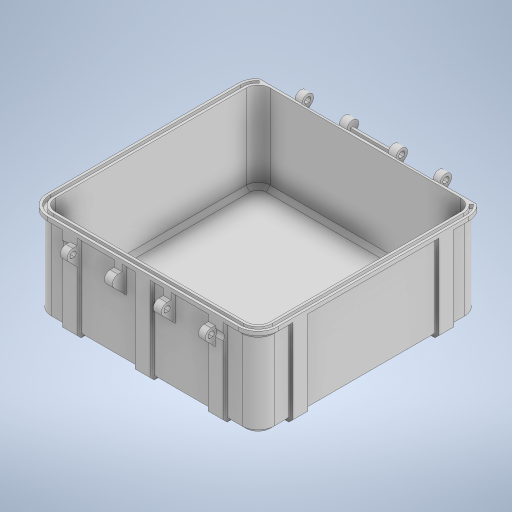
# Autodesk Inventor part: universal_box-main_body
Saved by Autodesk Inventor 2024 (Build 280153000, 153)
## iProperties
Created: 2024-03-05
Part Number: universal_box-main_body
Material: Všeobecné
Document SubType Name: Modeling
Designer: Simak
Density: 1 g/cm^3
Appearance: Výchozí
Author: Simak
Autodesk Inventor part; units mm, degrees
ref_plane "YZ Plane" through (0, 0, 0) normal (1, 0, 0) x (0, 1, 0)
ref_plane "XZ Plane" through (0, 0, 0) normal (0, 1, 0) x (-1, 0, 0)
ref_plane "XY Plane" through (0, 0, 0) normal (0, 0, 1) x (1, 0, 0)
sketch "velikost" plane through (0, 0, 0) normal (0, 1, 0) x (-1, 0, 0)
  line L0 (55.5, -55.5) -> (-55.5, -55.5)
  line L1 (-55.5, -55.5) -> (-55.5, 55.5)
  line L2 (-55.5, 55.5) -> (55.5, 55.5)
  line L3 (55.5, 55.5) -> (55.5, -55.5)
  line L4 (55.5, -55.5) -> (0, 0) construction
  line L5 (0, 0) -> (-55.5, -55.5) construction
  line L6 (0, 0) -> (-55.5, 55.5) construction
  dimension "d0" = 111
  dimension "d1" = 111
  constraints: 14 end point, 2 equal length, 2 parallel, 1 horizontal, 1 perpendicular
  measures "d0" distance of L0.start L0.end
  measures "d1" distance of L0.end L1.end
extrude "vyska" add sketch "velikost" along normal blind 46
fillet "Zaobleni_rohu" radius 8 4 edges at (-55.5, 23, 55.5) (55.5, 23, 55.5) (55.5, 23, -55.5) (-55.5, 23, -55.5)
shell "tloustka_sten" thickness 2 removed faces 1 at (15.8333, 46, -18.5)
sketch "vyztuhy-velikost" plane through (0, 46, 0) normal (0, 1, 0) x (1, 0, 0)
  arc A0 (-47.5, 53.5) -> (-53.5, 47.5) centre (-47.5, 47.5) ccw projected
  line L0 (-47.5, 53.5) -> (47.5, 53.5) projected
  arc A1 (53.5, 47.5) -> (47.5, 53.5) centre (47.5, 47.5) ccw projected
  line L1 (53.5, 47.5) -> (53.5, -47.5) projected
  arc A2 (47.5, -53.5) -> (53.5, -47.5) centre (47.5, -47.5) ccw projected
  line L2 (47.5, -53.5) -> (-47.5, -53.5) projected
  arc A3 (-53.5, -47.5) -> (-47.5, -53.5) centre (-47.5, -47.5) ccw projected
  line L3 (-53.5, -47.5) -> (-53.5, 47.5) projected
  arc A4 (-47.5, 55.5) -> (-55.5, 47.5) centre (-47.5, 47.5) ccw projected
  line L4 (-55.5, 47.5) -> (-55.5, -47.5) projected
  arc A5 (-55.5, -47.5) -> (-47.5, -55.5) centre (-47.5, -47.5) ccw projected
  line L5 (-47.5, -55.5) -> (47.5, -55.5) projected
  arc A6 (47.5, -55.5) -> (55.5, -47.5) centre (47.5, -47.5) ccw projected
  line L6 (55.5, -47.5) -> (55.5, 47.5) projected
  arc A7 (55.5, 47.5) -> (47.5, 55.5) centre (47.5, 47.5) ccw projected
  line L7 (47.5, 55.5) -> (-47.5, 55.5) projected
  line L8 (-40.1, 55.5) -> (-40.1, 57.5)
  line L9 (-40.1, 57.5) -> (-32.7, 57.5)
  line L10 (-32.7, 57.5) -> (-32.7, 55.5)
  line L11 (-3.7, 55.5) -> (-3.7, 57.5)
  line L12 (-3.7, 57.5) -> (3.7, 57.5)
  line L13 (3.7, 57.5) -> (3.7, 55.5)
  line L14 (32.7, 55.5) -> (32.7, 57.5)
  line L15 (32.7, 57.5) -> (40.1, 57.5)
  line L16 (40.1, 57.5) -> (40.1, 55.5)
  line L17 (47.5, 55.5) -> (-47.5, 55.5) projected
  line L18 (-3.7, 57.5) -> (0, 55.5) construction
  line L19 (3.7, 57.5) -> (0, 55.5) construction
  line L20 (-32.7, 57.5) -> (-3.7, 57.5) construction
  line L21 (3.7, 57.5) -> (32.7, 57.5) construction
  line L22 (-40.1, 57.5) -> (-47.5, 57.5) construction
  line L23 (-47.5, 57.5) -> (-47.5, 55.5) construction
  line L24 (-53.5, 0) -> (53.5, 0)
  line L25 (0, 53.5) -> (0, -53.5)
  line L26 (47.5, -53.5) -> (-47.5, -53.5) projected
  line L27 (-55.5, -40.1) -> (-57.5, -40.1)
  line L28 (-57.5, -40.1) -> (-57.5, -32.7)
  line L29 (-57.5, -32.7) -> (-55.5, -32.7)
  line L30 (-55.5, 32.7) -> (-57.5, 32.7)
  line L31 (-57.5, 32.7) -> (-57.5, 40.1)
  line L32 (-57.5, 40.1) -> (-55.5, 40.1)
  line L33 (-57.5, -32.7) -> (-57.5, 32.7) construction
  line L34 (-57.5, -40.1) -> (-57.5, -47.5) construction
  line L35 (-57.5, -47.5) -> (-55.5, -47.5) construction
  line L36 (-55.5, 47.5) -> (-55.5, -47.5) projected
  line L37 (-57.5, 40.1) -> (-57.5, 47.5) construction
  line L38 (-57.5, 47.5) -> (-55.5, 47.5) construction
  line L39 (-55.5, 0) -> (-57.5, 32.7) construction
  line L40 (-55.5, 0) -> (-57.5, -32.7) construction
  line L41 (-40.1, -55.5) -> (-40.1, -57.5)
  line L42 (-40.1, -57.5) -> (-32.7, -57.5)
  line L43 (-32.7, -57.5) -> (-32.7, -55.5)
  line L44 (-3.7, -55.5) -> (-3.7, -57.5)
  line L45 (-3.7, -57.5) -> (3.7, -57.5)
  line L46 (3.7, -57.5) -> (3.7, -55.5)
  line L47 (32.7, -55.5) -> (32.7, -57.5)
  line L48 (32.7, -57.5) -> (40.1, -57.5)
  line L49 (40.1, -57.5) -> (40.1, -55.5)
  line L50 (47.5, -55.5) -> (-47.5, -55.5)
  line L51 (-3.7, -57.5) -> (0, -55.5) construction
  line L52 (3.7, -57.5) -> (0, -55.5) construction
  line L53 (-32.7, -57.5) -> (-3.7, -57.5) construction
  line L54 (3.7, -57.5) -> (32.7, -57.5) construction
  line L55 (-40.1, -57.5) -> (-47.5, -57.5) construction
  line L56 (-47.5, -57.5) -> (-47.5, -55.5) construction
  line L57 (55.5, 47.5) -> (55.5, -47.5)
  line L58 (57.5, -32.7) -> (57.5, 32.7) construction
  line L59 (55.5, -40.1) -> (57.5, -40.1)
  line L60 (57.5, -40.1) -> (57.5, -47.5) construction
  line L61 (57.5, -32.7) -> (55.5, -32.7)
  line L62 (57.5, -47.5) -> (55.5, -47.5) construction
  line L63 (57.5, -40.1) -> (57.5, -32.7)
  line L64 (57.5, 32.7) -> (57.5, 40.1)
  line L65 (57.5, 40.1) -> (55.5, 40.1)
  line L66 (55.5, 32.7) -> (57.5, 32.7)
  line L67 (55.5, 47.5) -> (55.5, -47.5)
  line L68 (57.5, 40.1) -> (57.5, 47.5) construction
  line L69 (57.5, 47.5) -> (55.5, 47.5) construction
  line L70 (55.5, 0) -> (57.5, 32.7) construction
  line L71 (55.5, 0) -> (57.5, -32.7) construction
  point P0 (0, 0)
  point P1 (55.5, 40.1)
  point P2 (55.5, 32.7)
  point P3 (55.5, -32.7)
  point P4 (55.5, -40.1)
  point P5 (40.1, -55.5)
  point P6 (32.7, -55.5)
  point P7 (3.7, -55.5)
  point P8 (-3.7, -55.5)
  point P9 (-32.7, -55.5)
  point P10 (-40.1, -55.5)
  point P11 (-55.5, -40.1)
  point P12 (-55.5, -32.7)
  point P13 (-55.5, 32.7)
  point P14 (-55.5, 40.1)
  dimension "d6" = 2
  dimension "d7" = 7.4
  dimension "d8" = 2
  constraints: 120 end point, 25 symmetric about line, 20 point on line, 14 equal length, 11 perpendicular, 5 midpoint, 5 vertical, 2 horizontal, 5 other
  measures "d6" distance of L9.end L10.end
  measures "d7" distance of L11.end L12.end
  measures "d8" distance of L33.start L29.end
extrude "vyztuhy" add sketch "vyztuhy-velikost" against normal up to surface (46 mm away) contours L8 L9 L10 L7 | L4 L30 L31 L32 | L11 L12 L13 L7 | L4 L27 L28 L29 | L14 L15 L16 L7 | L5 L43 L42 L41 | L65 L64 L66 L6 | L5 L46 L45 L44 | L61 L63 L59 L6 | L5 L49 L48 L47
chamfer "Zkoseni_spodku" distance 2 angle 45 36 edges at (-18.2, 0, 55.5) (18.2, 0, 55.5) (0, 0, 57.5) (36.4, 0, 57.5) (43.8, 0, 55.5) (53.1569, 0, 53.1569) (55.5, 0, 43.8) (57.5, 0, 36.4) (55.5, 0, 0) (57.5, 0, -36.4) (53.1569, 0, -53.1569) (43.8, 0, -55.5) (55.5, 0, -43.8) (36.4, 0, -57.5) (18.2, 0, -55.5) (0, 0, -57.5) (-18.2, 0, -55.5) (-36.4, 0, -57.5) (-43.8, 0, -55.5) (-53.1569, 0, -53.1569) (-55.5, 0, -43.8) (-57.5, 0, -36.4) (-55.5, 0, 0) (-57.5, 0, 36.4) (-55.5, 0, 43.8) (-53.1569, 0, 53.1569) (-43.8, 0, 55.5) (-36.4, 0, 57.5) (-53.5, 2, 0) (-51.7426, 2, 51.7426) (0, 2, 53.5) (51.7426, 2, 51.7426) (53.5, 2, 0) (51.7426, 2, -51.7426) (0, 2, -53.5) (-51.7426, 2, -51.7426)
sketch "Náčrt4" plane through (40.1, 46, -55.5) normal (1, 0, 0) x (0, 0, -1)
  line L0 (-2, 0) -> (-2, -42) projected
  line L1 (2, 0) -> (2, -44) projected
  line L2 (-8, 0) -> (0, 0) projected
  line L3 (-0.75, 0) -> (-0.75, -2)
  line L4 (-0.75, -2) -> (0.75, -2)
  line L5 (0.75, -2) -> (0.75, 0)
  line L6 (-0.75, -2) -> (-2, -2) construction
  line L7 (0.75, -2) -> (2, -2) construction
  line L8 (2, 0) -> (0, 0) projected
  line L9 (2, -4) -> (-2, -4)
  point P0 (-55.5, -46)
  dimension "d16" = 1.5
  dimension "d17" = 2
  dimension "d18" = 2
  constraints: 12 end point, 7 point on line, 5 perpendicular, 1 collinear
  measures "d16" distance of L3.end L4.end
  measures "d17" distance between parallel lines of L8 L4
  measures "d18" distance between parallel lines of L9 L4
sketch "Náčrt3" plane through (0, 46, 0) normal (0, 1, 0) x (1, 0, 0)
  arc A0 (-47.5, 53.5) -> (-53.5, 47.5) centre (-47.5, 47.5) ccw projected
  line L0 (-47.5, 53.5) -> (47.5, 53.5) projected
  arc A1 (53.5, 47.5) -> (47.5, 53.5) centre (47.5, 47.5) ccw projected
  line L1 (53.5, 47.5) -> (53.5, -47.5) projected
  arc A2 (47.5, -53.5) -> (53.5, -47.5) centre (47.5, -47.5) ccw projected
  line L2 (47.5, -53.5) -> (-47.5, -53.5) projected
  arc A3 (-53.5, -47.5) -> (-47.5, -53.5) centre (-47.5, -47.5) ccw projected
  line L3 (-53.5, -47.5) -> (-53.5, 47.5) projected
  arc A4 (-47.5, 55.5) -> (-55.5, 47.5) centre (-47.5, 47.5) ccw projected
  line L4 (-55.5, 47.5) -> (-55.5, 40.1) projected
  line L5 (-57.5, 32.7) -> (-55.5, 32.7) projected
  line L6 (-55.5, 32.7) -> (-55.5, -32.7) projected
  arc A5 (-55.5, -47.5) -> (-47.5, -55.5) centre (-47.5, -47.5) ccw projected
  line L7 (-47.5, -55.5) -> (-40.1, -55.5) projected
  line L8 (-40.1, -55.5) -> (-40.1, -57.5) projected
  line L9 (-40.1, -57.5) -> (-32.7, -57.5) projected
  line L10 (-32.7, -57.5) -> (-32.7, -55.5) projected
  line L11 (-32.7, -55.5) -> (-3.7, -55.5) projected
  line L12 (-3.7, -55.5) -> (-3.7, -57.5) projected
  line L13 (-3.7, -57.5) -> (3.7, -57.5) projected
  line L14 (3.7, -57.5) -> (3.7, -55.5) projected
  line L15 (3.7, -55.5) -> (32.7, -55.5) projected
  line L16 (32.7, -55.5) -> (32.7, -57.5) projected
  line L17 (32.7, -57.5) -> (40.1, -57.5) projected
  line L18 (40.1, -57.5) -> (40.1, -55.5) projected
  line L19 (40.1, -55.5) -> (47.5, -55.5) projected
  arc A6 (47.5, -55.5) -> (55.5, -47.5) centre (47.5, -47.5) ccw projected
  line L20 (55.5, -47.5) -> (55.5, -40.1) projected
  line L21 (57.5, -32.7) -> (55.5, -32.7) projected
  line L22 (55.5, -32.7) -> (55.5, 32.7) projected
  arc A7 (55.5, 47.5) -> (47.5, 55.5) centre (47.5, 47.5) ccw projected
  line L23 (47.5, 55.5) -> (40.1, 55.5) projected
  line L24 (40.1, 55.5) -> (40.1, 57.5) projected
  line L25 (40.1, 57.5) -> (32.7, 57.5) projected
  line L26 (32.7, 57.5) -> (32.7, 55.5) projected
  line L27 (32.7, 55.5) -> (3.7, 55.5) projected
  line L28 (3.7, 55.5) -> (3.7, 57.5) projected
  line L29 (3.7, 57.5) -> (-3.7, 57.5) projected
  line L30 (-3.7, 57.5) -> (-3.7, 55.5) projected
  line L31 (-3.7, 55.5) -> (-32.7, 55.5) projected
  line L32 (-32.7, 55.5) -> (-32.7, 57.5) projected
  line L33 (-32.7, 57.5) -> (-40.1, 57.5) projected
  line L34 (-40.1, 57.5) -> (-40.1, 55.5) projected
  line L35 (-40.1, 55.5) -> (-47.5, 55.5) projected
  line L36 (-55.5, -32.7) -> (-57.5, -32.7) projected
  line L37 (-57.5, -32.7) -> (-57.5, -40.1) projected
  line L38 (55.5, 32.7) -> (57.5, 32.7) projected
  line L39 (57.5, 32.7) -> (57.5, 40.1) projected
  line L40 (-55.5, 40.1) -> (-57.5, 40.1) projected
  line L41 (-57.5, 40.1) -> (-57.5, 32.7) projected
  line L42 (-57.5, -40.1) -> (-55.5, -40.1) projected
  line L43 (-55.5, -40.1) -> (-55.5, -47.5) projected
  line L44 (55.5, -40.1) -> (57.5, -40.1) projected
  line L45 (57.5, -40.1) -> (57.5, -32.7) projected
  line L46 (57.5, 40.1) -> (55.5, 40.1) projected
  line L47 (55.5, 40.1) -> (55.5, 47.5) projected
  point P0 (0, 0)
sweep "tesnici_drazka" add profiles "Náčrt4" path "Náčrt3" path curves L0 A0 L3 A3 L2 A2 L1 A1 contours L2 L3 L4 L5 L8 L1 L9 L0
sweep "tesnici_drazka-zahloubeni" cut profiles "Náčrt4" path "Náčrt3" path curves L0 A0 L3 A3 L2 A2 L1 A1 contours L2 L8 L5 L4 L3
chamfer "tesnici_drazka-zkoseni" distance 2 angle 45 18 edges at (54.5711, 42, -54.5711) (43.8, 42, -57.5) (57.5, 42, -43.8) (18.2, 42, -57.5) (-18.2, 42, -57.5) (57.5, 42, 0) (57.5, 42, 43.8) (54.5711, 42, 54.5711) (43.8, 42, 57.5) (-54.5711, 42, -54.5711) (-57.5, 42, -43.8) (-43.8, 42, -57.5) (-57.5, 42, 0) (-54.5711, 42, 54.5711) (-43.8, 42, 57.5) (-57.5, 42, 43.8) (18.2, 42, 57.5) (-18.2, 42, 57.5)
sketch "pant-main_nacrt" plane through (32.7, 0, -55.5) normal (-1, 0, 0) x (0, 0, 1)
  line L0 (0, 2) -> (0, 42) projected
  line L1 (2, 0) -> (0, 2) projected
  line L2 (0, 0) -> (2, 0) projected
  line L3 (-2, 2) -> (0, 0) projected
  line L4 (-2, 44) -> (-2, 2) projected
  line L5 (0, 42) -> (-2, 44) projected
  circle A0 centre (-2, 46) radius 1.55
  circle A1 centre (-2, 46) radius 2.875
  line L6 (-4.0329, 43.9671) -> (-2, 41.9341)
  line L7 (-2, 41.9341) -> (0, 39.9341)
  line L8 (8, 44) -> (-2, 44) projected
  line L9 (8, 46) -> (8, 44) projected
  line L10 (-2, 46) -> (8, 46) projected
  line L11 (-2, 46) -> (-2, 44) projected
  line L12 (8, 42) -> (8, 44) projected
  line L13 (8, 44) -> (-2, 44) projected
  line L14 (0, 42) -> (-2, 44) projected
  line L15 (8, 42) -> (0, 42) projected
  line L16 (0.75, 44) -> (0.75, 46) projected
  line L17 (0.75, 44) -> (8, 44) projected
  line L18 (8, 44) -> (8, 46) projected
  line L19 (0.75, 46) -> (8, 46) projected
  line L20 (2, 46) -> (2, 4) projected
  circle A2 centre (-2, 46) radius 3.025
  circle A3 centre (-2, 46) radius 2.7
  point P0 (55.5, 0)
  point P1 (-2, 30)
  point P2 (0.875, 46)
  point P3 (-2, 43.125)
  point P4 (-1.23, 43.23)
  point P5 (0.0653, 44)
  point P6 (-2, 44)
  point P7 (-0.45, 46)
  point P8 (-2, 44.45)
  point P9 (0.75, 44.7398)
  point P10 (1.025, 46)
  point P11 (-1.1092, 43.1092)
  point P12 (-2, 42.975)
  point P13 (0.2695, 44)
  dimension "d28" = 5.75
  dimension "d27" = 3.1
  dimension "d71" = 0.15
  dimension "d78" = 5.4
  constraints: 4 end point, 3 centre point, 3 coincident, 2 point on line, 1 collinear, 1 parallel, 4 other
  measures "d27" diameter of A0
  measures "d78" diameter of A3
extrude "Vysunutí3" cut sketch "pant-main_nacrt" along normal blind 22 and the other way blind 3.5 contours A2 L4 A1 L5 | L5 A1 L8 A2 | A2 L6 A1 L4 | A2 L10 A1 L6 | A1 L4 A3 L5 | L5 A3 L8 A1 | L8 A1 L16 A2 | A1 L10 A3 L4 | A2 L16 A1 L10 | A3 L4 L5 | L5 L8 A3 | L8 A3 L10 L16 A1 | A3 L10 A0 L11 L4 | A1 L16 L10 | L11 A0 L10 A3 L8 | L11 L10 A0 | A0 L10 L11
extrude "Vysunutí18" cut sketch "pant-main_nacrt" against normal through all contours A3 L4 L5 | L5 L8 A3 | A3 L10 A0 L11 L4 | L11 A0 L10 A3 L8 | L11 L10 A0 | A0 L10 L11
extrude "Vysunutí4" add sketch "pant-main_nacrt" against normal blind 3.5 contours L6 A2 L4 | A2 L4 A1 L5 | L5 A1 L8 A2 | A2 L6 A1 L4 | A1 L4 A3 L5 | L5 A3 L8 A1 | A2 L16 L8 | L8 A1 L16 A2 | A1 L10 A3 L4 | A2 L16 A1 L10 | A3 L4 L5 | L5 L8 A3 | L8 A3 L10 L16 A1 | A3 L10 A0 L11 L4 | A1 L16 L10 | L11 A0 L10 A3 L8
extrude "Vysunutí19" add sketch "pant-main_nacrt" along normal up to surface (32.7 mm away) contours A2 L16 L8
sketch "Náčrt13" plane through (32.7, 0, -55.5) normal (-1, 0, 0) x (0, 0, 1)
  circle A0 centre (-2, 46) radius 1.55 projected
  line L0 (0.75, 46) -> (0.875, 46) projected
  line L1 (0.75, 44) -> (0.75, 46) projected
  line L2 (-0.1862, 44) -> (0.75, 44) projected
  arc A1 (-2, 43.3) -> (-0.1862, 44) centre (-2, 46) ccw projected
  line L3 (-2, 41.9341) -> (-2, 43.3) projected
  line L4 (-2, 41.9341) -> (-4.0329, 43.9671) projected
  arc A2 (0.875, 46) -> (-4.0329, 43.9671) centre (-2, 46) ccw projected
  line L5 (-2.75, 44.6435) -> (-2.75, 44.8)
  line L6 (-2.75, 44.8) -> (-1.25, 44.8)
  line L7 (-1.25, 44.8) -> (-1.25, 44.6435)
  point P0 (55.5, 0)
  dimension "d83" = 2.75
  dimension "d84" = 1.5
  constraints: 6 end point, 2 perpendicular, 2 point on circle, 1 parallel, 1 vertical
  measures "d84" distance of L5.end L6.end
extrude "Vysunutí20" add sketch "Náčrt13" against normal up to surface (3.5 mm away) contours L5 L6 L7 A0 picked at (-2.0521, 44.686)
ref_plane "Pracovní rovina1" through (14.2, 0, -55.5) normal (-1, 0, 0) x (0, 0, 1)
sketch "Náčrt14" plane through (14.2, 0, -55.5) normal (-1, 0, 0) x (0, 0, 1)
  arc A0 (-1.1092, 43.1092) -> (1.025, 46) centre (-2, 46) ccw projected
  line L0 (1.025, 46) -> (0.875, 46) projected
  arc A1 (0.875, 46) -> (-4.0329, 43.9671) centre (-2, 46) ccw projected
  line L1 (-4.0329, 43.9671) -> (-2, 41.9341) projected
  line L2 (-2, 41.9341) -> (-2, 2) projected
  line L3 (0, 0) -> (-2, 2) projected
  line L4 (2, 0) -> (0, 0) projected
  line L5 (0, 2) -> (2, 0) projected
  line L6 (0, 42) -> (0, 2) projected
  line L7 (-1.1092, 43.1092) -> (0, 42) projected
  arc A2 (-1.25, 44.6435) -> (-2.75, 44.6435) centre (-2, 46) ccw projected
  line L8 (-1.25, 44.6435) -> (-1.25, 44.8) projected
  line L9 (-1.25, 44.8) -> (-2.75, 44.8) projected
  line L10 (-2.75, 44.8) -> (-2.75, 44.6435) projected
  line L11 (-2, 41.9341) -> (0, 39.9341)
  point P0 (55.5, 0)
  constraints: 2 end point, 1 collinear, 1 point on line
extrude "Vysunutí21" add sketch "Náčrt14" along normal up to surface (3.5 mm away) contours L7 L6 L11 L1 A1 L0 A0
sketch "Náčrt15" plane through (10.7, 39.9341, -55.5) normal (-1, 0, 0) x (0, 0, 1)
  line L0 (0.875, 6.0659) -> (0.75, 6.0659) projected
  arc A0 (0.875, 6.0659) -> (-4.0329, 4.0329) centre (-2, 6.0659) ccw projected
  line L1 (0, 0) -> (-4.0329, 4.0329) projected
  line L2 (-2, 4.8659) -> (-2, 4.0659) projected
  line L3 (-2.75, 4.8659) -> (-2, 4.8659) projected
  line L4 (-2.75, 4.7094) -> (-2.75, 4.8659) projected
  arc A1 (-0.75, 5.1493) -> (-2.75, 4.7094) centre (-2, 6.0659) ccw projected
  line L5 (-0.75, 4.0659) -> (-0.75, 5.1493) projected
  line L6 (0.2695, 4.0659) -> (-0.75, 4.0659) projected
  line L7 (0.75, 6.0659) -> (0.75, 4.8057) projected
  arc A2 (-1.1092, 3.175) -> (1.025, 6.0659) centre (-2, 6.0659) ccw projected
  line L8 (-1.1092, 3.175) -> (0, 2.0659) projected
  arc A3 (0.2695, 4.0659) -> (0.75, 4.8057) centre (-2, 6.0659) ccw projected
  line L9 (0, 2.0659) -> (0, 0) projected
  line L10 (-2, 4.0659) -> (0, 2.0659) projected
  point P0 (55.5, -39.9341)
  point P1 (0.2695, 4.0659)
  point P2 (0.75, 4.8057)
extrude "Vysunutí22" add sketch "Náčrt15" along normal blind 0.5 contours L0 L7 A2 L6 L5 A1 L4 L3 L2 L10 L8 L9 L1 A0
sketch "Náčrt16" plane through (32.7, 2, -55.5) normal (0, 0, -1) x (-1, 0, 0)
  line L0 (18.5, 41.1092) -> (18.5, 44) projected
  line L1 (0, 44) -> (18.5, 44) projected
  line L2 (0, 44) -> (0, 41.1092) projected
  line L3 (18.5, 41.1092) -> (0, 41.1092) projected
  line L4 (18.5, 41.1092) -> (0, 41.1092) projected
  line L5 (0, 41.1092) -> (0, 40) projected
  line L6 (18.5, 40) -> (0, 40) projected
  line L7 (22.5, 37.9341) -> (18.5, 37.9341) projected
  line L8 (18.5, 40) -> (0, 40) projected
  line L9 (0, 40) -> (0, 0) projected
  line L10 (29, 0) -> (0, 0) projected
  line L11 (29, 0) -> (29, 40) projected
  line L12 (65.4, 40) -> (36.4, 40) projected
  line L13 (36.4, 40) -> (36.4, 0) projected
  line L14 (65.4, 0) -> (36.4, 0) projected
  line L15 (65.4, 0) -> (65.4, 40) projected
  line L16 (18.5, 40) -> (18.5, 41.1092) projected
  line L17 (18.5, 37.9341) -> (18.5, 40) projected
  line L18 (22.5, 40) -> (22.5, 37.9341) projected
  line L19 (29, 40) -> (22.5, 40) projected
  point P0 (32.7, -2)
extrude "Vysunutí23" cut sketch "Náčrt16" along normal through all contours L3 L2 L1 L0 | L16 L6 L5 L3
sketch "Náčrt17" plane through (36.2, 0, -55.5) normal (1, 0, 0) x (0, 0, -1)
  arc A0 (2.75, 44.6435) -> (1.25, 44.6435) centre (2, 46) ccw projected
  line L0 (2.75, 44.6435) -> (2.75, 44.8) projected
  line L1 (2.75, 44.8) -> (1.25, 44.8) projected
  line L2 (1.25, 44.8) -> (1.25, 44.6435) projected
  line L3 (-0.75, 46) -> (-0.875, 46) projected
  line L4 (-0.75, 44) -> (-0.75, 46) projected
  line L5 (0.1862, 44) -> (-0.75, 44) projected
  arc A1 (0.1862, 44) -> (2, 43.3) centre (2, 46) ccw projected
  line L6 (2, 41.9341) -> (2, 43.3) projected
  line L7 (2, 41.9341) -> (4.0329, 43.9671) projected
  arc A2 (4.0329, 43.9671) -> (-0.875, 46) centre (2, 46) ccw projected
  spline S0 degree 6 poles (0.1863, 43.9999) (0.1273, 44.0533) (0.0685, 44.1105) (0.0102, 44.1714) (-0.0473, 44.2362) (-0.1036, 44.305) (-0.193, 44.4239) (-0.227, 44.4717) (-0.2603, 44.521) (-0.2927, 44.5719) (-0.3241, 44.6243) (-0.3771, 44.7188) (-0.3992, 44.7602) (-0.4207, 44.8024) (-0.4414, 44.8454) (-0.4613, 44.8891) (-0.5499, 45.0952) (-0.6084, 45.266) (-0.6538, 45.4443) (-0.6846, 45.6278) (-0.7, 45.814) (-0.7, 46) knots 0 0 0 0 0 0 0 0.258993 0.258993 0.258993 0.258993 0.258993 0.423699 0.423699 0.423699 0.423699 0.423699 0.547895 0.547895 0.547895 0.547895 0.547895 1 1 1 1 1 1 1 projected
  line L8 (-0.7, 46) -> (-8, 46) projected
  point P0 (-55.5, 0)
  constraints: 1 other
extrude "Vysunutí24" add sketch "Náčrt17" along normal up to next contours L8 S0 L5 L4
sketch "Náčrt18" plane through (0, 46, 0) normal (0, 1, 0) x (1, 0, 0)
  arc A0 (56.25, 47.5) -> (52.399, 54.75) centre (47.5, 47.5) ccw projected
  arc A1 (54.75, 47.5) -> (47.5, 54.75) centre (47.5, 47.5) ccw projected
  line L0 (47.5, 47.5) -> (53.3577, 54)
  line L1 (47.5, 54.75) -> (52.399, 54.75) projected
  line L2 (54.3345, 54.8) -> (36.2, 54.8) projected
  point P0 (0, 0)
  point P1 (52.3535, 52.8857)
  dimension "d99" = 0.8
  constraints: 2 end point, 1 point on circle
  measures "d99" distance from line of L2 L0.end
extrude "Vysunutí25" add sketch "Náčrt18" against normal up to next
sketch "Náčrt19" plane through (10.7, 0, -55.5) normal (1, 0, 0) x (0, 0, -1)
  arc A0 (4.0329, 43.9671) -> (-0.875, 46) centre (2, 46) ccw projected
  line L0 (-1.025, 46) -> (-0.875, 46) projected
  arc A1 (-1.025, 46) -> (0, 43.7305) centre (2, 46) ccw projected
  line L1 (4.0329, 43.9671) -> (0, 39.9341) projected
  arc A2 (2.75, 44.6435) -> (1.25, 44.6435) centre (2, 46) ccw projected
  line L2 (2.75, 44.8) -> (2.75, 44.6435) projected
  line L3 (1.25, 44.8) -> (2.75, 44.8) projected
  line L4 (1.25, 44.6435) -> (1.25, 44.8) projected
  line L5 (0, 39.9341) -> (0, 43.7305) projected
  point P0 (-55.5, 0)
extrude "Vysunutí26" add sketch "Náčrt19" against normal up to surface (0.5 mm away) contours L2 L3 L4 A2
mirror "pant-zrcadleni" about plane through (0, 0, 0) normal (1, 0, 0) of "Vysunutí3", "Vysunutí4", "Vysunutí24", "Vysunutí25", "Vysunutí23", "Vysunutí22", "Vysunutí21", "Vysunutí19", "Vysunutí20", "Vysunutí18", "Vysunutí26"
sketch "latch-main_nacrt" plane through (32.7, 0, 53.5) normal (-1, 0, 0) x (0, 0, 1)
  line L0 (4, 44) -> (4, 2) projected
  line L1 (2, 0) -> (4, 2) projected
  line L2 (0, 0) -> (2, 0) projected
  line L3 (2, 2) -> (0, 0) projected
  line L4 (2, 42) -> (2, 2) projected
  line L5 (4, 44) -> (2, 42) projected
  line L6 (4, 46) -> (-6, 46) projected
  line L7 (2.75, 44) -> (-6, 44) projected
  line L8 (1.25, 44) -> (1.25, 46) projected
  line L9 (2.75, 44) -> (2.75, 46) projected
  line L10 (4, 46) -> (4, 44) projected
  circle A0 centre (6.05, 37.8) radius 1.55
  line L11 (5.3, 36.4435) -> (5.3, 36.6)
  line L12 (5.3, 36.6) -> (6.8, 36.6)
  line L13 (6.8, 36.6) -> (6.8, 36.4435)
  circle A1 centre (6.05, 37.8) radius 2.875
  line L14 (6.05, 40.675) -> (2, 40.675)
  line L15 (2, 29.6841) -> (8.0829, 35.7671)
  circle A2 centre (6.05, 37.8) radius 2.7
  point P0 (-53.5, 0)
  point P1 (4, 39.8157)
  point P2 (4, 35.7843)
  dimension "d52" = 3.1
  dimension "d53" = 8.2
  dimension "d54" = 4.05
  dimension "d55" = 2.75
  dimension "d56" = 1.5
  dimension "d57" = 5.75
  dimension "d58" = 45
  dimension "d63" = 5.4
  constraints: 10 end point, 4 point on circle, 3 centre point, 3 perpendicular, 2 coincident, 2 point on line, 2 tangent, 1 parallel, 1 vertical
  measures "d52" diameter of A0
  measures "d53" distance from line of L6 A0.centre
  measures "d54" distance from line of L4 A0.centre
  measures "d56" distance of L11.end L12.end
  measures "d57" diameter of A1
  measures "d58" angle of L4 L15
  measures "d63" diameter of A2
extrude "Vysunutí14" cut sketch "latch-main_nacrt" against normal up to next contours A2 L0 | L0 A2
extrude "Vysunutí12" add sketch "latch-main_nacrt" against normal blind 3.5 contours L14 A1 L0 | L0 A1 L15 L4 L14 | A1 L0 A2 | L0 A2 A1 | A2 L0 | L0 A2 | A1 L15 L0 | L11 L12 L13 A0 picked at (5.9979, 36.486)
ref_plane "Pracovní rovina3" through (14.2, 0, 53.5) normal (-1, 0, 0) x (0, 0, 1)
sketch "Náčrt10" plane through (14.2, 0, 53.5) normal (-1, 0, 0) x (0, 0, 1)
  arc A0 (6.8, 36.4435) -> (5.3, 36.4435) centre (6.05, 37.8) ccw projected
  line L0 (6.8, 36.4435) -> (6.8, 36.6) projected
  line L1 (6.8, 36.6) -> (5.3, 36.6) projected
  line L2 (5.3, 36.6) -> (5.3, 36.4435) projected
  line L3 (4, 31.6841) -> (8.0829, 35.7671) projected
  arc A1 (8.0829, 35.7671) -> (6.05, 40.675) centre (6.05, 37.8) ccw projected
  line L4 (6.05, 40.675) -> (4, 40.675) projected
  line L5 (4, 44) -> (4, 40.675) projected
  line L6 (2, 42) -> (4, 44) projected
  line L7 (2, 2) -> (2, 42) projected
  line L8 (0, 0) -> (2, 2) projected
  line L9 (2, 0) -> (0, 0) projected
  line L10 (4, 2) -> (2, 0) projected
  line L11 (4, 31.6841) -> (4, 2) projected
  line L12 (4, 40.675) -> (2, 40.675)
  line L13 (4, 31.6841) -> (2, 29.6841)
  line L14 (4, 40.675) -> (2, 42)
  point P0 (-53.5, 0)
  constraints: 6 end point, 2 collinear, 2 point on line
extrude "Vysunutí15" add sketch "Náčrt10" along normal blind 4 contours L13 L7 L12 L4 A1 L3 | L7 L14 L12 | L14 L6 L5
sketch "Náčrt12" plane through (10.2, 0, 53.5) normal (-1, 0, 0) x (0, 0, 1)
  line L0 (2, 29.6841) -> (8.0829, 35.7671) projected
  arc A0 (8.0829, 35.7671) -> (6.05, 40.675) centre (6.05, 37.8) ccw projected
  line L1 (6.05, 40.675) -> (4, 40.675) projected
  line L2 (6.8, 36.6) -> (5.3, 36.6) projected
  line L3 (5.3, 36.6) -> (5.3, 36.4435) projected
  arc A1 (6.8, 36.4435) -> (5.3, 36.4435) centre (6.05, 37.8) ccw projected
  line L4 (6.8, 36.4435) -> (6.8, 36.6) projected
  line L5 (4, 40.675) -> (4, 44) projected
  line L6 (2, 42) -> (4, 44) projected
  line L7 (2, 29.6841) -> (2, 42) projected
  point P0 (-53.5, 0)
extrude "Vysunutí16" add sketch "Náčrt12" against normal blind 0.5 contours L2 L3 A1 L4
mirror "latch-zrcadleni" about plane through (0, 0, 0) normal (1, 0, 0) of "Vysunutí16", "Vysunutí14", "Vysunutí12", "Vysunutí15"
fillet "Zaoblení2" radius 1 8 edges at (43.8, 43.3736, -56.8737) (50.4352, 43.4845, -56.519) (54.0393, 44.8323, -55.0656) (38.15, 43.3, -57.5) (-38.15, 43.3, -57.5) (-50.4352, 43.4845, -56.519) (-43.8, 43.3736, -56.8737) (-54.0393, 44.8323, -55.0656)
ref_plane "Pracovní rovina2" through (-14.2, 0, -55.5) normal (-1, 0, 0) x (0, 0, 1)
ref_plane "Pracovní rovina4" through (-14.2, 0, 53.5) normal (-1, 0, 0) x (0, 0, 1)
